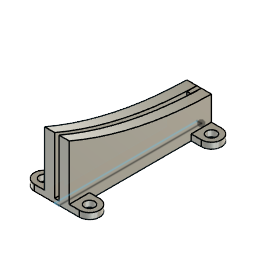
Wire Cutter Stand (Autodesk Fusion 360 design; units mm, degrees)
part number: 2025-10-17-09-51-47-009
Autodesk Fusion 360 part; units mm, degrees
sketch "Sketch1" plane through (0, 0, 0) normal (1, 0, 0) x (0, 1, 0)
  line L0 (-35, 15) -> (-35, -15)
  line L1 (-35, -15) -> (35, -15)
  line L2 (35, -15) -> (35, 0)
  line L3 (35, 15) -> (-35, -15) construction
  line L4 (-35, 15) -> (35, -15) construction
  arc A0 (-35, 15) -> (35, 0) centre (38.2143, 185.8333) ccw
  dimension "d1" = 70
  dimension "d2" = 30
  constraint parallel L0 L2
  constraint coincident L3 origin
  constraint coincident L4 origin
  constraint tangent L4 A0
  measures "d2" distance of L0.start L0.end
extrude "Extrude1" add sketch "Sketch1" along normal blind 5 makes body 1
ref_plane "WorkPlane1" through (-10, 0, 0) normal (-1, 0, 0) x (0, -1, 0)
sketch "Sketch2" plane through (0, 0, 0) normal (0, 0, 1) x (1, 0, 0)
ref_plane "WorkPlane2" through (0, 0, -15) normal (0, 0, 1) x (1, 0, 0)
sketch "Sketch3" plane through (0, 0, -15) normal (0, 0, 1) x (1, 0, 0)
  circle A0 centre (10, 30) radius 2.5
  arc A1 (15, 30) -> (10, 35) centre (10, 30) ccw
  line L0 (5, 35) -> (10, 35)
  arc A2 (10, 25) -> (15, 30) centre (10, 30) ccw
  line L1 (10, 25) -> (5, 25)
  arc A3 (10, -35) -> (15, -30) centre (10, -30) ccw
  line L2 (5, -25) -> (5, -35)
  line L3 (5, 25) -> (5, 35)
  arc A4 (15, -30) -> (10, -25) centre (10, -30) ccw
  line L4 (5, -35) -> (10, -35)
  circle A5 centre (10, -30) radius 2.5
  line L5 (10, -25) -> (5, -25)
  dimension "d13" = 5
  dimension "d14" = 5
  dimension "d15" = 5
  dimension "d16" = 5
  dimension "d17" = 5
  dimension "d18" = 5
  constraint horizontal L4
  constraint horizontal L5
  constraint vertical L2
  constraint horizontal L0
  constraint horizontal L1
  constraint vertical L3
  constraint tangent A3 L4
  constraint concentric A3 A5
  constraint tangent A2 L1
  constraint tangent A4 L5
  constraint coincident A3.end A4.start
  constraint tangent A1 L0
  constraint coincident A1.start A2.end
  measures "d13" radius of A3
  measures "d14" diameter of A5
  measures "d15" diameter of A0
  measures "d16" radius of A2
  measures "d17" radius of A4
  measures "d18" radius of A1
extrude "Extrude2" add sketch "Sketch3" along normal blind 3 bodies 1
mirror "Mirror1" about plane through (-10, 0, 0) normal (-1, 0, 0) of bodies 1 makes body 2
move_body "Move1" bodies 2 to x (1, 0, 0) y (0, 1, 0) z (0, 0, 1) at (8.75, 0, 0)
move_body "Move2" bodies 1 to x (1, 0, 0) y (0, 1, 0) z (0, 0, 1) at (-8.75, 0, 0)
move_body "Move3" bodies 2 to x (1, 0, 0) y (0, 1, 0) z (0, 0, 1) at (0.15, 0, 0)
move_body "Move4" bodies 1 to x (1, 0, 0) y (0, 1, 0) z (0, 0, 1) at (-0.15, 0, 0)
move_body "Move5" bodies 2 to x (1, 0, 0) y (0, 1, 0) z (0, 0, 1) at (0.05, 0, 0)
move_body "Move6" bodies 1 to x (1, 0, 0) y (0, 1, 0) z (0, 0, 1) at (-0.05, 0, 0)
move_body "Move7" bodies 2 to x (1, 0, 0) y (0, 1, 0) z (0, 0, 1) at (-0.025, 0, 0)
move_body "Move8" bodies 1 to x (1, 0, 0) y (0, 1, 0) z (0, 0, 1) at (0.025, 0, 0)
sketch "Sketch4" plane through (0, 0, -15) normal (0, 0, -1) x (1, 0, 0)
  circle A0 centre (1.075, 30) radius 2.5
  circle A1 centre (1.075, -30) radius 2.5
  line L0 (-8.925, 35) -> (-8.925, -35)
  line L1 (-8.925, -35) -> (1.075, -35)
  arc A2 (1.075, -35) -> (1.075, -25) centre (1.075, -30) ccw
  line L2 (1.075, -25) -> (-3.925, -25)
  line L3 (-3.925, -25) -> (-3.925, 25)
  line L4 (-3.925, 25) -> (1.075, 25)
  arc A3 (1.075, 25) -> (1.075, 35) centre (1.075, 30) ccw
  line L5 (1.075, 35) -> (-8.925, 35)
  line L6 (-8.925, -35) -> (-11, -35)
  line L7 (-11, -35) -> (-11, 35)
  line L8 (-11, 35) -> (-8.925, 35)
  line L9 (-8.925, 35) -> (-8.925, -35)
  constraint horizontal L6
  constraint vertical L7
  constraint horizontal L8
  constraint vertical L9
  constraint coincident L0.end L1.start
sketch "Sketch5" plane through (0, 0, -15) normal (0, 0, -1) x (1, 0, 0)
  line L0 (-8, -35) -> (-12, -35)
  line L1 (-12, -35) -> (-12, 35)
  line L2 (-12, 35) -> (-8, 35)
  line L3 (-8, 35) -> (-8, -35)
  constraint horizontal L0
  constraint vertical L1
  constraint horizontal L2
  constraint vertical L3
extrude "Extrude3" add sketch "Sketch5" against normal blind 2 bodies 1 2
sketch "Sketch6" plane through (-16.075, 0, 0) normal (-1, 0, 0) x (0, -1, 0)
  line L0 (25, -15) -> (25, -12)
  line L1 (25, -12) -> (35, -12)
  line L2 (35, -12) -> (35, 15)
  arc A0 (-35, 0) -> (35, 15) centre (-38.2143, 185.8333) ccw
  line L3 (-35, 0) -> (-35, -12)
  line L4 (-35, -12) -> (-25, -12)
  line L5 (-25, -12) -> (-25, -15)
  line L6 (-25, -15) -> (25, -15)
  line L7 (-35, 0) -> (-30, 0)
  line L8 (-30, 0) -> (-30, -15)
  line L9 (-30, -15) -> (-35, -15)
  line L10 (-35, -15) -> (-35, 0)
  constraint horizontal L7
  constraint vertical L8
  constraint horizontal L9
  constraint vertical L10
  constraint coincident A0.start L3.start
extrude "Extrude4" add sketch "Sketch6" against normal blind 11 contours L4 L8 L9 L10 | L3 L4 L7 L8 L10 bodies 1
sketch "Sketch7" plane through (-16.075, 0, 0) normal (-1, 0, 0) x (0, -1, 0)
  line L0 (-35, -12) -> (-25, -12)
  line L1 (-25, -12) -> (-25, -15)
  line L2 (-25, -15) -> (25, -15)
  line L3 (25, -15) -> (25, -12)
  line L4 (25, -12) -> (35, -12)
  line L5 (35, -12) -> (35, 15)
  arc A0 (-35, 0) -> (35, 15) centre (-38.2143, 185.8333) ccw
  line L6 (-35, 0) -> (-35, -12)
equation "d23 = 10.00 mm - 1.25 mm"
equation "d26 = -10 mm + 1.25 mm"
